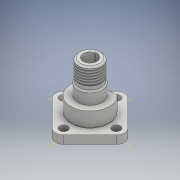
# Autodesk Inventor part: 1
Saved by Autodesk Inventor 2018 (Build 220112000, 112)
## iProperties
Created: 2020-05-28
Part Number: 1
Material: Типовые
Document SubType Name: Modeling
Designer: 2000
Density: 1 g/cm^3
Appearance: По умолчанию
Author: 2000
Autodesk Inventor part; units mm, degrees
ref_plane "YZ Plane" through (0, 0, 0) normal (1, 0, 0) x (0, 1, 0)
ref_plane "XZ Plane" through (0, 0, 0) normal (0, 1, 0) x (-1, 0, 0)
ref_plane "XY Plane" through (0, 0, 0) normal (0, 0, 1) x (1, 0, 0)
sketch "Эскиз1" plane through (0, 0, 0) normal (0, 0, 1) x (1, 0, 0)
  line L0 (10.6066, 58.6899) -> (58.6899, 10.6066)
  line L1 (58.6899, -10.6066) -> (10.6066, -58.6899)
  line L2 (-10.6066, -58.6899) -> (-58.6899, -10.6066)
  line L3 (-58.6899, 10.6066) -> (-10.6066, 58.6899)
  circle A0 centre (0, 48.0833) radius 7.5
  circle A1 centre (48.0833, 0) radius 7.5
  circle A2 centre (0, -48.0833) radius 7.5
  circle A3 centre (-48.0833, 0) radius 7.5
  arc A4 (10.6066, 58.6899) -> (-10.6066, 58.6899) centre (0, 48.0833) ccw
  arc A5 (58.6899, -10.6066) -> (58.6899, 10.6066) centre (48.0833, 0) ccw
  arc A6 (-10.6066, -58.6899) -> (10.6066, -58.6899) centre (0, -48.0833) ccw
  arc A7 (-58.6899, 10.6066) -> (-58.6899, -10.6066) centre (-48.0833, 0) ccw
  line L4 (-97.0151, 0) -> (97.0151, 0) projected
  line L5 (0, -97.0151) -> (0, 97.0151) projected
  point P0 (0, 69.2965)
  point P1 (69.2965, 0)
  point P2 (0, -69.2965)
  point P3 (-69.2965, 0)
  dimension "d4" = 15
  dimension "d5" = 15
  dimension "d6" = 15
  dimension "d7" = 15
  dimension "d8" = 68
  dimension "d10" = 68
  dimension "d16" = 15
  dimension "d21" = 68
  dimension "d22" = 98
  dimension "d23" = 98
  dimension "d25" = 68
  dimension "d26" = 96.1665
  constraints: 14 point on line, 8 centre point, 8 end point, 8 point on circle, 8 tangent, 3 equal radius, 2 parallel, 1 horizontal alignment, 1 perpendicular
  measures "d4" diameter of A2
  measures "d5" diameter of A0
  measures "d6" diameter of A1
  measures "d7" diameter of A3
  measures "d8" distance of A1.centre A0.centre
  measures "d10" distance of A1.centre A2.centre
  measures "d16" radius of A4
  measures "d21" distance of A3.centre A2.centre
  measures "d22" distance between parallel lines of L0 L2
  measures "d23" distance between parallel lines of L1 L3
  measures "d25" distance of A3.centre A0.centre
  measures "d26" distance of A2.centre A0.centre
extrude "Выдавливание1" add sketch "Эскиз1" along normal blind 15 contours L0 A5 L4 A1 L5 A0 A4 | L5 A0 L4 A3 A7 L3 A4 | A5 L1 A6 L5 A2 L4 A1 | L4 A3 L5 A2 A6 L2 A7
sketch "Эскиз2" plane through (0, 0, 15) normal (0, 0, 1) x (1, 0, 0)
  circle A0 centre (0, 0) radius 34
  dimension "d29" = 68
  constraints: 1 centre point, 1 coincident
  measures "d29" diameter of A0
extrude "Выдавливание2" add sketch "Эскиз2" along normal blind 2
sketch "Эскиз3" plane through (0, 0, 17) normal (0, 0, 1) x (1, 0, 0)
  circle A0 centre (0, 0) radius 35
  dimension "d32" = 70
  constraints: 1 centre point, 1 coincident
  measures "d32" diameter of A0
extrude "Выдавливание3" add sketch "Эскиз3" along normal blind 26
sketch "Эскиз4" plane through (0, 0, 43) normal (0, 0, 1) x (1, 0, 0)
  circle A0 centre (0, 0) radius 35 projected
  line L0 (-24.4949, 25) -> (24.4949, 25)
  dimension "d35" = 25
  constraints: 2 end point, 2 point on circle, 1 horizontal
  measures "d35" distance from line of point (0, 0) L0
extrude "Выдавливание4" cut sketch "Эскиз4" against normal blind 26 contours L0 A0 picked at (6.1349, 26.5901)
sketch "Эскиз5" plane through (0, 0, 43) normal (0, 0, 1) x (1, 0, 0)
  circle A0 centre (0, 0) radius 22.5
  dimension "d38" = 45
  constraints: 1 centre point, 1 coincident
  measures "d38" diameter of A0
extrude "Выдавливание5" add sketch "Эскиз5" along normal blind 20
sketch "Эскиз6" plane through (0, 0, 63) normal (0, 0, 1) x (1, 0, 0)
  circle A0 centre (0, 0) radius 20.25
  dimension "d41" = 40.5
  constraints: 1 centre point, 1 coincident
  measures "d41" diameter of A0
extrude "Выдавливание6" add sketch "Эскиз6" along normal blind 10
sketch "Эскиз7" plane through (0, 0, 73) normal (0, 0, 1) x (1, 0, 0)
  circle A0 centre (0, 0) radius 21
  dimension "d44" = 42
  constraints: 1 centre point, 1 coincident
  measures "d44" diameter of A0
extrude "Выдавливание7" add sketch "Эскиз7" along normal blind 30
sketch "Эскиз8" plane through (0, 0, 0) normal (0, 0, -1) x (-1, 0, 0)
  circle A0 centre (0, 0) radius 25
  dimension "d47" = 50
  constraints: 1 centre point, 1 coincident
  measures "d47" diameter of A0
extrude "Выдавливание8" cut sketch "Эскиз8" against normal blind 5
sketch "Эскиз9" plane through (0, 0, 103) normal (0, 0, 1) x (1, 0, 0)
  arc A0 (-3, 12.1347) -> (3, 12.1347) centre (0, 0) ccw
  line L0 (3, 12.1347) -> (3, 13.5)
  line L1 (3, 13.5) -> (-3, 13.5)
  line L2 (-3, 13.5) -> (-3, 12.1347)
  line L3 (0, -88.3166) -> (0, 88.3166) projected
  dimension "d51" = 25
  dimension "d52" = 6
  dimension "d54" = 13.5
  dimension "d55" = 6
  constraints: 6 end point, 2 point on circle, 1 centre point, 1 coincident, 1 parallel, 1 other
  measures "d51" diameter of A0
  measures "d52" distance of L0.end L1.end
  measures "d54" distance from line of point (0, 0) L1
  measures "d55" distance between parallel lines of L0 L2
extrude "Выдавливание9" cut sketch "Эскиз9" against normal blind 103
sketch "Эскиз10" plane through (0, 0, 5) normal (0, 0, -1) x (-1, 0, 0)
  circle A0 centre (0, 0) radius 15
  dimension "d58" = 30
  constraints: 1 centre point, 1 coincident
  measures "d58" diameter of A0
extrude "Выдавливание10" cut sketch "Эскиз10" against normal blind 40
fillet "Сопряжение2" radius 1 1 edges at (-20.25, 0, 73)
fillet "Сопряжение3" radius 3 1 edges at (-20.25, 0, 63)
thread "Резьба1" size "M42x4.5" class "6g" standard "ANSI Metric M Profile" full length
chamfer "Фаска1" distance 3 angle 45 1 edges at (-21, 0, 103)
